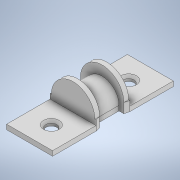
# Autodesk Inventor part: SUPPORT_POULIE_ARRIERE
Saved by Autodesk Inventor 2020 (Build 240168000, 168)
## iProperties
Created: 2020-06-12
Part Number: SUPPORT_POULIE_ARRIERE
Material: Generic
Document SubType Name: Modeling
Designer: Admin
Density: 1 g/cm^3
Appearance: Default
Author: Admin
Autodesk Inventor part; units mm, degrees
ref_plane "YZ Plane" through (0, 0, 0) normal (1, 0, 0) x (0, 1, 0)
ref_plane "XZ Plane" through (0, 0, 0) normal (0, 1, 0) x (-1, 0, 0)
ref_plane "XY Plane" through (0, 0, 0) normal (0, 0, 1) x (1, 0, 0)
sketch "Sketch1" plane through (0, 0, 0) normal (0, 1, 0) x (-1, 0, 0)
  line L0 (0, 0) -> (19, 0)
  line L1 (19, 0) -> (19, -50)
  line L2 (19, -50) -> (0, -50)
  line L3 (0, -50) -> (0, 0)
  dimension "d0" = 50
  dimension "d1" = 19
  constraints: 8 end point, 2 parallel, 1 horizontal, 1 perpendicular
  measures "d0" distance of L0.end L1.end
  measures "d1" distance of L1.end L2.end
extrude "Extrusion1" add sketch "Sketch1" along normal blind 2
sketch "Sketch2" plane through (0, 2, 0) normal (0, 1, 0) x (1, 0, 0)
  line L0 (-19, 20) -> (-16.5, 20)
  line L1 (-16.5, 20) -> (-16.5, 30)
  line L2 (-16.5, 30) -> (-19, 30)
  line L3 (-19, 30) -> (-19, 20)
  line L4 (-19, 0) -> (0, 0) projected
  line L5 (-19, 50) -> (-19, 0) projected
  line L6 (-2.5, 20) -> (0, 20)
  line L7 (0, 20) -> (0, 30)
  line L8 (0, 30) -> (-2.5, 30)
  line L9 (-2.5, 30) -> (-2.5, 20)
  line L10 (0, 0) -> (0, 50) projected
  dimension "d4" = 2.5
  dimension "d5" = 10
  dimension "d6" = 20
  dimension "d7" = 10
  dimension "d8" = 2.5
  dimension "d9" = 20
  constraints: 16 end point, 4 parallel, 2 horizontal, 2 perpendicular, 2 point on line
  measures "d4" distance of L1.end L2.end
  measures "d5" distance of L2.end L0.start
  measures "d6" distance from line of L4 L0.start
  measures "d7" distance of L8.end L6.start
  measures "d8" distance of L7.end L8.end
  measures "d9" distance between parallel lines of L4 L6
extrude "Extrusion2" cut sketch "Sketch2" against normal through all
sketch "Sketch3" plane through (-16.5, 2, -20) normal (0, 0, -1) x (-1, 0, 0)
  line L0 (2.5, 0) -> (-16.5, 0) projected
  arc A0 (0, 0) -> (-14, 0) centre (-7, 0) ccw
  point P0 (-16.5, -2)
  dimension "d12" = 7
  constraints: 2 point on circle, 1 centre point
  measures "d12" radius of A0
extrude "Extrusion3" add sketch "Sketch3" along normal blind 10
sketch "Sketch5" plane through (0, 2, 0) normal (0, 1, 0) x (1, 0, 0)
  line L0 (-16.5, 20) -> (-19, 20) projected
  line L1 (-19, 20) -> (0, 20)
  line L2 (0, 20) -> (0, 18)
  line L3 (0, 18) -> (-19, 18)
  line L4 (-19, 18) -> (-19, 20)
  line L5 (-19, 30) -> (-16.5, 30) projected
  line L6 (-19, 30) -> (0, 30)
  line L7 (0, 30) -> (0, 32)
  line L8 (0, 32) -> (-19, 32)
  line L9 (-19, 32) -> (-19, 30)
  line L10 (0, 0) -> (0, 20) projected
  line L11 (0, 30) -> (0, 50) projected
  dimension "d15" = 2
  dimension "d16" = 2
  constraints: 16 end point, 4 parallel, 2 horizontal, 2 perpendicular, 2 point on line
  measures "d15" distance of L8.end L5.start
  measures "d16" distance of L3.end L0.end
extrude "Extrusion4" add sketch "Sketch5" along normal blind 2
sketch "Sketch6" plane through (-16.5, 2, -30) normal (0, 0, -1) x (-1, 0, 0)
  arc A0 (2, 2) -> (-16, 2) centre (-7, 2) ccw
  line L0 (2.5, 0) -> (2.5, 2) projected
  line L1 (-13.7082, 2) -> (-0.2918, 2) projected
  line L2 (2, 2) -> (-16, 2)
  point P0 (-16.5, -2)
  dimension "d19" = 9
  dimension "d21" = 0
  dimension "d22" = 0
  dimension "d23" = 9.5
  dimension "d24" = 0
  constraints: 2 end point, 2 point on circle, 1 centre point
  measures "d19" radius of A0
  measures "d21" vertical distance of A0.centre L2.start
  measures "d22" vertical distance of A0.centre L2.end
  measures "d23" distance from line of A0.centre L0
  measures "d24" distance from line of L1 A0.centre
extrude "Extrusion5" add sketch "Sketch6" along normal blind 2
sketch "Sketch7" plane through (-16.5, 2, -20) normal (0, 0, 1) x (1, 0, 0)
  arc A0 (16, 2) -> (-2, 2) centre (7, 2) ccw
  line L0 (-2.5, 2) -> (16.5, 2) projected
  point P0 (16.5, -2)
  point P1 (7, 2)
  point P2 (-2, 2)
  point P3 (16, 2)
  dimension "d27" = 9
  dimension "d28" = 0
  dimension "d29" = 0
  constraints: 2 point on circle, 1 centre point, 1 coincident, 1 midpoint
  measures "d27" radius of A0
  measures "d28" vertical distance of A0.centre A0.end
  measures "d29" vertical distance of A0.start A0.centre
extrude "Extrusion6" add sketch "Sketch7" along normal blind 2
sketch "Sketch8" plane through (0, 4, 0) normal (0, 1, 0) x (1, 0, 0)
  line L0 (0, 18) -> (-19, 18) projected
  line L1 (-19, 20) -> (-16.5, 20) projected
  line L2 (-19, 18) -> (-19, 20)
  line L3 (-19, 20) -> (-18.5, 20)
  line L4 (-18.5, 20) -> (-19, 18)
  line L5 (-0.5, 30) -> (-18.5, 30) projected
  line L6 (-19, 50) -> (-19, 32) projected
  line L7 (-18.5, 30) -> (-19, 32)
  line L8 (-19, 32) -> (-19, 30)
  line L9 (-19, 30) -> (-18.5, 30)
  line L10 (0, 20) -> (-0.5, 20) projected
  line L11 (-0.5, 20) -> (0, 20)
  line L12 (0, 18) -> (0, 20) projected
  line L13 (0, 20) -> (0, 18)
  line L14 (0, 18) -> (-0.5, 20)
  line L15 (0, 30) -> (-2.5, 30) projected
  line L16 (0, 30) -> (0, 32) projected
  line L17 (0, 32) -> (0, 30)
  line L18 (0, 30) -> (-0.5, 30)
  line L19 (-0.5, 32) -> (-0.5, 30) projected
  line L20 (-0.5, 30) -> (0, 32)
  point P0 (0, 0)
  constraints: 24 end point, 3 collinear, 3 perpendicular, 1 horizontal, 1 parallel, 1 point on line
extrude "Extrusion7" cut sketch "Sketch8" against normal through all
sketch "Sketch9" plane through (0, 2, 0) normal (0, 1, 0) x (1, 0, 0)
  circle A0 centre (-9.5, 9) radius 2.25
  circle A1 centre (-9.5, 41) radius 2.25
  line L0 (-19, 0) -> (0, 0) projected
  line L1 (0, 50) -> (-19, 50) projected
  line L2 (-19, 18) -> (-19, 0) projected
  line L3 (-19, 50) -> (-19, 32) projected
  dimension "d34" = 4.5
  dimension "d35" = 4.5
  dimension "d36" = 9
  dimension "d37" = 9
  dimension "d38" = 9.5
  dimension "d39" = 9.5
  constraints: 2 centre point
  measures "d34" diameter of A0
  measures "d35" diameter of A1
  measures "d36" distance from line of L0 A0.centre
  measures "d37" distance from line of L1 A1.centre
  measures "d38" distance from line of L2 A0.centre
  measures "d39" distance from line of L3 A1.centre
extrude "Extrusion8" cut sketch "Sketch9" against normal through all
chamfer "Chamfer1" distance 1 angle 45 2 edges at (-11.75, 2, -9) (-11.75, 2, -41)
body "Solid1"
